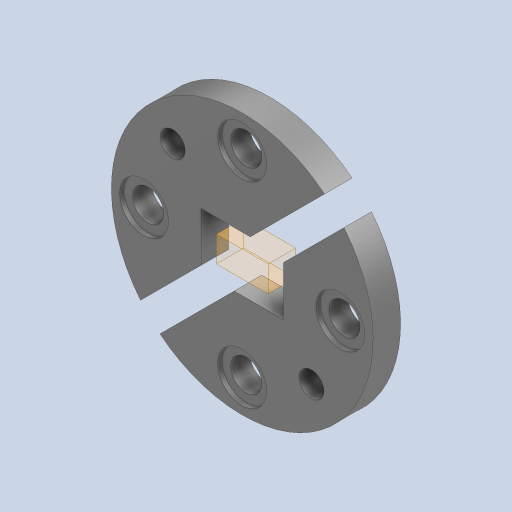
# Autodesk Inventor part: RWG-V_Band Backingplate
Saved by Autodesk Inventor 2023.2 (Build 272271000, 271)
## iProperties
Created: 2024-09-19
Part Number: RWG-V_Band Backingplate
Material: Generisch
Document SubType Name: Modeling
Designer: Nils Bade
Density: 1 g/cm^3
Appearance: Vorgabe
Author: Nils Bade
Autodesk Inventor part; units mm, degrees
ref_plane "YZ Plane" through (0, 0, 0) normal (1, 0, 0) x (0, 1, 0)
ref_plane "XZ Plane" through (0, 0, 0) normal (0, 1, 0) x (-1, 0, 0)
sketch "S-Flansch" plane through (0, 0, 0) normal (0, 0, 1) x (1, 0, 0)
  circle A0 centre (0, 0) radius 9.525
  circle A1 centre (0, 0) radius 7.144 construction
  circle A2 centre (0, 7.144) radius 1.1305
  circle A3 centre (0, 7.144) radius 1.778
  line L0 (0, 0) -> (5.0516, 5.0516) construction
  line L1 (0, 13.335) -> (0, -13.335) construction
  circle A4 centre (5.0516, 5.0516) radius 0.9
  circle A5 centre (-7.144, 0) radius 1.1305
  circle A6 centre (-7.144, 0) radius 1.778
  circle A7 centre (-5.0516, 5.0516) radius 0.9
  circle A8 centre (0, -7.144) radius 1.1305
  circle A9 centre (0, -7.144) radius 1.778
  circle A10 centre (-5.0516, -5.0516) radius 0.9
  circle A11 centre (7.144, 0) radius 1.1305
  circle A12 centre (7.144, 0) radius 1.778
  circle A13 centre (5.0516, -5.0516) radius 0.9
  line L2 (-3, 2) -> (3, 2)
  line L3 (3, 2) -> (3, -2)
  line L4 (3, -2) -> (-3, -2)
  line L5 (-3, -2) -> (-3, 2)
  line L6 (-3, 2) -> (3, -2) construction
  line L7 (3, 2) -> (-3, -2) construction
  line L8 (-1.8795, 0.94) -> (1.8795, 0.94)
  line L9 (1.8795, 0.94) -> (1.8795, -0.94)
  line L10 (1.8795, -0.94) -> (-1.8795, -0.94)
  line L11 (-1.8795, -0.94) -> (-1.8795, 0.94)
  line L12 (-1.8795, 0.94) -> (1.8795, -0.94) construction
  line L13 (1.8795, 0.94) -> (-1.8795, -0.94) construction
  dimension "d0" = 19.05
  dimension "d1" = 14.288
  dimension "d2" = 2.261
  dimension "d3" = 3.556
  dimension "d4" = 45
  dimension "d5" = 1.8
  dimension "d8" = 360
  dimension "d10" = 6
  dimension "d11" = 4
  dimension "d16" = 3.759
  dimension "d17" = 1.88
  constraints: 26 end point, 14 centre point, 7 coincident, 4 midpoint, 4 parallel, 2 horizontal, 2 perpendicular, 2 point on circle, 1 point on line, 25 other
  measures "d0" diameter of A0
  measures "d1" diameter of A1
  measures "d2" diameter of A2
  measures "d3" diameter of A3
  measures "d4" angle of L1 L0
  measures "d5" diameter of A4
  measures "d10" distance between parallel lines of L5 L3
  measures "d11" distance between parallel lines of L4 L2
  measures "d16" distance of L8.start L8.end
  measures "d17" distance between parallel lines of L8 L10
extrude "Ex-Flansch1" add sketch "S-Flansch" along normal mid plane 2 contours A0
ref_plane "Schnittebene" through (0.7071, -0.7071, 0) normal (0.7071068, -0.7071068, 0) x (0.7071068, 0.7071068, 0)
ref_plane "Querebene" through (0, 0, 0) normal (0.7071068, -0.7071068, 0) x (0.7071068, 0.7071068, 0)
split "Trennen-Schnitt" plane through (0.7071, -0.7071, 0) removes the side toward (-0.7071068, 0.7071068, 0)
extrude "Ex-Flansch2-Innengewinde" add sketch "S-Flansch" along normal mid plane 1.4 contours A9 | A12
pattern_circular "Runde Anordnung1" count 2 over 360 about axis through (0, 0, -10) along (0, 0, 1)
surface extrude "RWG-V-Band" sketch "S-Flansch" along normal mid plane 2 shown yes curves L9 L10 L11 L8
